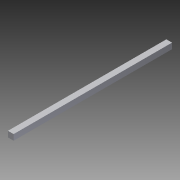
# Autodesk Inventor part: Cremaillere
Saved by Autodesk Inventor 2014 SP1 (Build 180222100, 222)
## iProperties
Created: 2015-05-01
Part Number: Cremaillere
Material: PPS Plastic
Document SubType Name: Modeling
Designer: david
Density: 1.637 g/cm^3
Appearance: Smooth - White
Mass: 33.1493 g
Surface Area: 91.62 cm^2
Volume: 20.25 cm^3
Author: david
Autodesk Inventor part; units mm, degrees
ref_plane "YZ Plane" through (0, 0, 0) normal (1, 0, 0) x (0, 1, 0)
ref_plane "XZ Plane" through (0, 0, 0) normal (0, 1, 0) x (-1, 0, 0)
ref_plane "XY Plane" through (0, 0, 0) normal (0, 0, 1) x (1, 0, 0)
sketch "Sketch1" plane through (0, 0, 0) normal (0, 1, 0) x (-1, 0, 0)
  line L0 (-4.5, 4.5) -> (4.5, 4.5)
  line L1 (4.5, 4.5) -> (4.5, -4.5)
  line L2 (4.5, -4.5) -> (-4.5, -4.5)
  line L3 (-4.5, -4.5) -> (-4.5, 4.5)
  line L4 (-4.5, 4.5) -> (4.5, -4.5) construction
  line L5 (4.5, 4.5) -> (-4.5, -4.5) construction
  point P0 (0, 0)
  dimension "d0" = 9
  dimension "d1" = 9
  constraints: 12 end point, 2 midpoint, 2 parallel, 1 horizontal, 1 perpendicular
  measures "d0" distance of L1.end L2.end
  measures "d1" distance of L0.end L1.end
extrude "Extrusion1" add sketch "Sketch1" along normal blind 250
body "Solid1"
